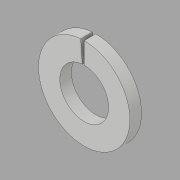
# Autodesk Inventor part: Washer - Split - 92146A029
Saved by Autodesk Inventor 2017 (Build 210142000, 142)
## iProperties
Created: 2022-08-16
Part Number: Washer - Split - 92146A029
Material: Generic
Document SubType Name: Modeling
Designer: JTS
Density: 1 g/cm^3
Appearance: Default
Author: JTS
Autodesk Inventor part; units mm, degrees
ref_plane "YZ Plane" through (0, 0, 0) normal (1, 0, 0) x (0, 1, 0)
ref_plane "XZ Plane" through (0, 0, 0) normal (0, 1, 0) x (-1, 0, 0)
ref_plane "XY Plane" through (0, 0, 0) normal (0, 0, 1) x (1, 0, 0)
sketch "Sketch1" plane through (0, 0, 0) normal (0, 0, 1) x (1, 0, 0)
  arc A0 (-0.4679, 6.1672) -> (0, 6.1849) centre (0, 0) ccw
  arc A1 (-0.2498, 3.2925) -> (0, 3.302) centre (0, 0) ccw
  line L0 (0, 0) -> (-0.2498, 3.2925) construction
  line L1 (0, 0) -> (0, 3.302) construction
  line L2 (-0.2498, 3.2925) -> (-0.4679, 6.1672)
  line L3 (0, 3.302) -> (0, 6.1849)
  dimension "d0" = 0.25
  dimension "d1" = 6.1849
  dimension "d2" = 3.302
  constraints: 8 end point, 4 point on circle, 2 centre point, 2 coincident, 2 collinear, 1 vertical
  measures "d0" distance of L1.end L0.end
  measures "d1" radius of A0
  measures "d2" radius of A1
extrude "Extrusion1" add sketch "Sketch1" along normal blind 1.5748
body "Solid1"
